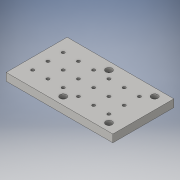
# Autodesk Inventor part: M605-to-X95-adapter-V1
Saved by Autodesk Inventor 2016 (Build 200138000, 138)
## iProperties
Created: 2018-06-26
Part Number: M605-to-X95-adapter-V1
Material: Generic
Document SubType Name: Modeling
Designer: voigt
Density: 1 g/cm^3
Appearance: Default
Author: voigt
Autodesk Inventor part; units mm, degrees
ref_plane "YZ Plane" through (0, 0, 0) normal (1, 0, 0) x (0, 1, 0)
ref_plane "XZ Plane" through (0, 0, 0) normal (0, 1, 0) x (-1, 0, 0)
ref_plane "XY Plane" through (0, 0, 0) normal (0, 0, 1) x (1, 0, 0)
sketch "Sketch1" plane through (0, 0, 0) normal (0, 0, 1) x (1, 0, 0)
  line L0 (0, 70) -> (0, -70) construction
  line L1 (-153.5, 0) -> (91.5, 0) construction
  line L2 (-118.5, 50) -> (56.5, 50)
  line L3 (56.5, 50) -> (56.5, -50)
  line L4 (56.5, -50) -> (-118.5, -50)
  line L5 (-118.5, -50) -> (-118.5, 50)
  point P0 (0, 0)
  dimension "d0" = 100
  dimension "d1" = 56.5
  dimension "d2" = 175
  constraints: 8 end point, 2 parallel, 1 horizontal, 1 perpendicular, 1 other
  measures "d0" distance between parallel lines of L4 L2
  measures "d1" distance between parallel lines of L3 L0
  measures "d2" distance between parallel lines of L5 L3
extrude "Extrusion1" add sketch "Sketch1" along normal blind 12.5
sketch "Sketch2" plane through (0, 0, 12.5) normal (0, 0, 1) x (1, 0, 0)
  line L0 (56.5, 50) -> (-118.5, 50) construction
  line L1 (-118.5, 50) -> (-118.5, -50) construction
  line L2 (-118.5, -50) -> (56.5, -50) construction
  line L3 (56.5, -50) -> (56.5, 50) construction
  line L4 (0, 70) -> (0, -70) construction
  line L5 (-153.5, 0) -> (91.5, 0) construction
  line L6 (-37.5, 37.5) -> (37.5, 37.5) construction
  line L7 (37.5, 37.5) -> (37.5, -37.5) construction
  line L8 (37.5, -37.5) -> (-37.5, -37.5) construction
  line L9 (-37.5, -37.5) -> (-37.5, 37.5) construction
  point P0 (0, 0)
  dimension "d5" = 75
  dimension "d6" = 75
  constraints: 8 end point, 4 coincident, 2 parallel, 1 horizontal, 1 perpendicular, 2 other
  measures "d5" distance between parallel lines of L8 L6
  measures "d6" distance between parallel lines of L9 L7
hole "Hole1" at (-37.5, 37.5, 12.5) at (-37.5, -37.5, 12.5) at (37.5, -37.5, 12.5) at (37.5, 37.5, 12.5) direction (0, 0, -1) diameter 6 end through all counterbore diameter 10.5 counterbore depth 7
sketch "Sketch3" plane through (0, 0, 12.5) normal (0, 0, 1) x (1, 0, 0)
  circle A0 centre (-37.5, -37.5) radius 5.25 construction
  circle A1 centre (-37.5, 37.5) radius 5.25 construction
  circle A2 centre (37.5, -37.5) radius 5.25 construction
  line L0 (56.5, 50) -> (-118.5, 50) construction
  line L1 (-118.5, 50) -> (-118.5, -50) construction
  line L2 (-118.5, -50) -> (56.5, -50) construction
  line L3 (56.5, -50) -> (56.5, 50) construction
  line L4 (-153.5, 0) -> (91.5, 0) construction
  line L5 (0, 70) -> (0, -70) construction
  point P0 (0, 0)
  point P1 (25, 25)
  point P2 (0, 25)
  point P3 (-25, 25)
  point P4 (-50, 25)
  point P5 (-75, 25)
  point P6 (-100, 25)
  point P7 (25, 0)
  point P8 (0, 0)
  point P9 (-25, 0)
  point P10 (-50, 0)
  point P11 (-75, 0)
  point P12 (-100, 0)
  point P13 (25, -25)
  point P14 (0, -25)
  point P15 (-25, -25)
  point P16 (-50, -25)
  point P17 (-75, -25)
  point P18 (-100, -25)
  dimension "d14" = 25
  dimension "d15" = 25
  dimension "d18" = 25
  dimension "d21" = 25
  constraints: 1 horizontal, 1 vertical, 17 other
  measures "d14" distance from line of L5 point (25, 25)
  measures "d15" distance from line of L4 point (25, 25)
  measures "d18" distance of point (25, 25) point (0, 25)
  measures "d21" distance of point (25, 25) point (25, 0)
hole "Hole2" at (0, 0, 12.5) at (25, 25, 12.5) at (0, 25, 12.5) at (-25, 25, 12.5) at (-50, 25, 12.5) at (-75, 25, 12.5) at (-100, 25, 12.5) at (25, 0, 12.5) at (-25, 0, 12.5) at (-50, 0, 12.5) at (-75, 0, 12.5) at (-100, 0, 12.5) at (25, -25, 12.5) at (0, -25, 12.5) at (-25, -25, 12.5) at (-50, -25, 12.5) at (-75, -25, 12.5) at (-100, -25, 12.5) direction (0, 0, -1) diameter 4.917 end through all thread size "M6x1" class "6H" standard "ANSI Metric M Profile"
body "Solid1"
